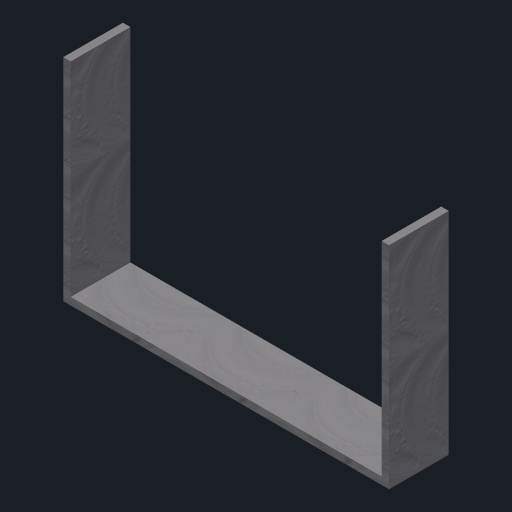
# Autodesk Inventor part: SOPORTE_METAL_PAP
Saved by Autodesk Inventor 2024.3 (Build 283343000, 343)
## iProperties
Created: 2024-07-25
Part Number: SOPORTE_METAL_PAP
Material: Steel, Mild, Welded
Document SubType Name: Modeling
Designer: Niler
Density: 7.85 g/cm^3
Appearance: Weld - Steel Mild
Author: Niler
Autodesk Inventor part; units mm, degrees
ref_plane "YZ Plane" through (0, 0, 0) normal (1, 0, 0) x (0, 1, 0)
ref_plane "XZ Plane" through (0, 0, 0) normal (0, 1, 0) x (-1, 0, 0)
ref_plane "XY Plane" through (0, 0, 0) normal (0, 0, 1) x (1, 0, 0)
sketch "Sketch1" plane through (0, 0, 0) normal (0, 0, 1) x (1, 0, 0)
  line L0 (-69.375, 0) -> (69.375, 0)
  line L1 (-69.375, 0) -> (-69.375, 90)
  line L2 (0, 0) -> (0, 9.6097)
  line L3 (69.375, 0) -> (69.375, 90)
  line L4 (66.2, 90) -> (66.2, 3.175)
  line L5 (66.2, 3.175) -> (-66.2, 3.175)
  line L6 (-66.2, 3.175) -> (-66.2, 90)
  line L7 (-69.375, 90) -> (-66.2, 90)
  line L8 (66.2, 90) -> (69.375, 90)
  dimension "d0" = 3.175
  dimension "d1" = 132.4
  dimension "d2" = 90
  dimension "d5" = 90
  constraints: 18 end point, 2 perpendicular, 1 coincident, 1 horizontal, 1 horizontal alignment, 1 midpoint, 1 symmetric about line, 1 vertical, 2 other
  measures "d0" distance between parallel lines of L0 L5
  measures "d1" distance of L4.start L6.end
  measures "d2" angle of L5 L6
  measures "d5" distance from line of L0 L4.start
extrude "Extrusion1" add sketch "Sketch1" along normal mid plane 25.4
body "Solid1"
